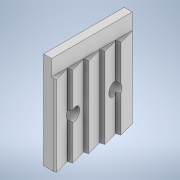
# Autodesk Inventor part: suporte estruzor 3
Saved by Autodesk Inventor 2022 (Build 260153000, 153)
## iProperties
Created: 2022-02-16
Part Number: suporte estruzor 3
Material: Genérico
Document SubType Name: Modeling
Designer: mathe
Density: 1 g/cm^3
Appearance: Padrão
Author: mathe
Autodesk Inventor part; units mm, degrees
ref_plane "YZ Plane" through (0, 0, 0) normal (1, 0, 0) x (0, 1, 0)
ref_plane "XZ Plane" through (0, 0, 0) normal (0, 1, 0) x (-1, 0, 0)
ref_plane "XY Plane" through (0, 0, 0) normal (0, 0, 1) x (1, 0, 0)
sketch "Esboço1" plane through (0, 0, 0) normal (0, 1, 0) x (-1, 0, 0)
  line L0 (84, 0) -> (82.9647, 3.8637)
  line L1 (82.9647, 3.8637) -> (84, 4.1411)
  line L2 (84, 4) -> (82.9647, 7.8637)
  line L3 (82.9647, 7.8637) -> (84, 8.1411)
  line L4 (84, 0) -> (84.9017, 0)
  line L5 (84, 0) -> (86, 0)
  line L6 (84, 8) -> (82.9647, 11.8637)
  line L7 (84, 24) -> (83.9647, 24.1317)
  line L8 (82.9647, 27.8637) -> (84, 28.1411)
  line L9 (84, 28) -> (82.9647, 31.8637)
  line L10 (82.9647, 31.8637) -> (84, 32.1411)
  line L11 (84, 32) -> (82.9647, 35.8637)
  line L12 (82.9647, 35.8637) -> (84, 36.1411)
  line L13 (84, 36) -> (82.9647, 39.8637)
  line L14 (82.9647, 39.8637) -> (84, 40.1411)
  line L15 (84, 0) -> (80, 0) construction
  line L16 (82.9647, 11.8637) -> (84, 12.1411)
  line L17 (84, 12) -> (82.9647, 15.8637)
  line L18 (82.9647, 15.8637) -> (84, 16.1411)
  line L19 (84, 16) -> (82.9647, 19.8637)
  line L20 (82.9647, 19.8637) -> (83.4734, 20)
  line L21 (83.9647, 24.1317) -> (84, 24.1411)
  line L22 (84, 0) -> (82.9647, 3.8637)
  line L23 (82.9647, 3.8637) -> (84, 4.1411)
  line L24 (84, 4) -> (82.9647, 7.8637)
  line L25 (82.9647, 7.8637) -> (84, 8.1411)
  line L26 (84, 0) -> (84.9017, 0)
  line L27 (84, 0) -> (86, 0)
  line L28 (84, 8) -> (82.9647, 11.8637)
  line L29 (84, 24) -> (83.9647, 24.1317)
  line L30 (82.9647, 27.8637) -> (84, 28.1411)
  line L31 (84, 28) -> (82.9647, 31.8637)
  line L32 (82.9647, 31.8637) -> (84, 32.1411)
  line L33 (84, 32) -> (82.9647, 35.8637)
  line L34 (82.9647, 35.8637) -> (84, 36.1411)
  line L35 (84, 36) -> (82.9647, 39.8637)
  line L36 (82.9647, 39.8637) -> (84, 40.1411)
  line L37 (84, 0) -> (80, 0) construction
  line L38 (82.9647, 11.8637) -> (84, 12.1411)
  line L39 (84, 12) -> (82.9647, 15.8637)
  line L40 (82.9647, 15.8637) -> (84, 16.1411)
  line L41 (84, 16) -> (82.9647, 19.8637)
  line L42 (82.9647, 19.8637) -> (83.4734, 20)
  line L43 (83.9647, 24.1317) -> (84, 24.1411)
  line L44 (84, 0) -> (86, 0)
  line L45 (86, 0) -> (86, 20)
  line L46 (86, 20) -> (84, 20)
  line L47 (84, 20) -> (84, 0)
  line L48 (84, 20) -> (83.4734, 20)
  point P0 (0, 0)
  point P1 (83.9647, 16.1317)
  point P2 (83.9647, 12.1317)
  point P3 (83.9647, 8.1317)
  point P4 (83.9647, 4.1317)
  constraints: 98 end point, 2 horizontal, 2 parallel, 2 point on line, 1 perpendicular
extrude "Extrusão1" add sketch "Esboço1" along normal blind 24 contours L47 L46 L45 L5 L4
extrude "Extrusão2" add sketch "Esboço1" along normal blind 20 contours L0 L1 L2 L47 | L2 L3 L6 L47 L1 | L6 L16 L17 L47 L3 | L47 L18 L19 L20 L48 | L17 L18 L19 L47 L16
sketch "Esboço2" plane through (-86, 0, 0) normal (-1, 0, 0) x (0, 0, 1)
  point P0 (0, 0)
  point P1 (5, 10)
  point P2 (15, 10)
hole "Furo1" at (-86, 10, 5) at (-86, 10, 15) direction (1, 0, 0) diameter 3 end through all
